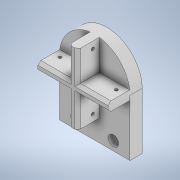
# Autodesk Inventor part: Test_Stand_Mounting_Plate
Saved by Autodesk Inventor 2022 (Build 260153000, 153)
## iProperties
Created: 2021-08-03
Part Number: Test_Stand_Mounting_Plate
Material: Generic
Document SubType Name: Modeling
Designer: exllu
Density: 1 g/cm^3
Appearance: Default
Author: exllu
Autodesk Inventor part; units mm, degrees
ref_plane "YZ Plane" through (0, 0, 0) normal (1, 0, 0) x (0, 1, 0)
ref_plane "XZ Plane" through (0, 0, 0) normal (0, 1, 0) x (-1, 0, 0)
ref_plane "XY Plane" through (0, 0, 0) normal (0, 0, 1) x (1, 0, 0)
sketch "Sketch1" plane through (0, 0, 0) normal (0, 0, 1) x (1, 0, 0)
  circle A0 centre (0, 0) radius 37.5
  line L0 (0, 0) -> (0, -25)
  circle A1 centre (0, -25) radius 3
  dimension "d0" = 75
  dimension "d1" = 25
  dimension "d2" = 6
  constraints: 2 centre point, 2 coincident, 2 end point, 1 vertical
  measures "d0" diameter of A0
  measures "d1" distance of L0.start L0.end
  measures "d2" diameter of A1
extrude "Extrusion1" add sketch "Sketch1" along normal blind 8 contours A0 | A1
sketch "Sketch2" plane through (0, 0, 8) normal (0, 0, 1) x (1, 0, 0)
  line L0 (0, 0) -> (17.6777, 17.6777)
  line L1 (0, 0) -> (25, 0) construction
  circle A0 centre (17.6777, 17.6777) radius 3.15
  circle A1 centre (-17.6777, 17.6777) radius 3.15
  circle A2 centre (-17.6777, -17.6777) radius 3.15
  circle A3 centre (17.6777, -17.6777) radius 3.15
  dimension "d5" = 25
  dimension "d6" = 45
  dimension "d7" = 6.3
  dimension "d10" = 360
  constraints: 4 centre point, 4 end point, 1 coincident, 1 equal length, 1 horizontal, 9 other
  measures "d5" distance of L0.start L0.end
  measures "d6" angle of L1 L0
  measures "d7" diameter of A0
extrude "Extrusion2" cut sketch "Sketch2" against normal blind 10
sketch "Sketch3" plane through (0, 0, 8) normal (0, 0, 1) x (1, 0, 0)
  arc A0 (-21.9203, 13.435) -> (-13.435, 21.9203) centre (-17.6777, 17.6777) ccw
  line L0 (-17.6777, 17.6777) -> (-11.6777, 17.6777) construction
  line L1 (-13.435, 21.9203) -> (-19.9189, 28.4042)
  line L2 (-21.9203, 13.435) -> (-28.4042, 19.9189)
  line L3 (-28.4042, 19.9189) -> (-19.9189, 28.4042)
  arc A1 (-13.435, -21.9203) -> (-21.9203, -13.435) centre (-17.6777, -17.6777) ccw
  line L4 (-17.6777, -17.6777) -> (-17.6777, -11.6777) construction
  line L5 (-21.9203, -13.435) -> (-28.4042, -19.9189)
  line L6 (-13.435, -21.9203) -> (-19.9189, -28.4042)
  line L7 (-19.9189, -28.4042) -> (-28.4042, -19.9189)
  arc A2 (21.9203, -13.435) -> (13.435, -21.9203) centre (17.6777, -17.6777) ccw
  line L8 (17.6777, -17.6777) -> (11.6777, -17.6777) construction
  line L9 (13.435, -21.9203) -> (19.9189, -28.4042)
  line L10 (21.9203, -13.435) -> (28.4042, -19.9189)
  line L11 (28.4042, -19.9189) -> (19.9189, -28.4042)
  arc A3 (13.435, 21.9203) -> (21.9203, 13.435) centre (17.6777, 17.6777) ccw
  line L12 (17.6777, 17.6777) -> (17.6777, 11.6777) construction
  line L13 (21.9203, 13.435) -> (28.4042, 19.9189)
  line L14 (13.435, 21.9203) -> (19.9189, 28.4042)
  line L15 (19.9189, 28.4042) -> (28.4042, 19.9189)
  circle A4 centre (0, 0) radius 31.5
  point P0 (-26.1087, 17.6234)
  point P1 (-26.1087, -17.6234)
  point P2 (-17.6234, -26.1087)
  point P3 (17.6234, -26.1087)
  point P4 (26.1087, -17.6234)
  point P5 (26.1087, 17.6234)
  point P6 (17.6234, 26.1087)
  point P7 (-17.6234, 26.1087)
  dimension "d14" = 12
  dimension "d18" = 360
  constraints: 32 end point, 8 point on circle, 5 centre point, 5 coincident, 2 tangent, 1 horizontal, 1 perpendicular, 49 other
  measures "d14" diameter of A0
sketch "Sketch4" plane through (0, 0, 0) normal (0, 0, -1) x (-1, 0, 0)
  circle A0 centre (0, 0) radius 42.8826
  constraints: 1 centre point, 1 coincident
extrude "Extrusion4" cut sketch "Sketch4" against normal blind 2
sketch "Sketch5" plane through (0, 0, 8) normal (0, 0, 1) x (1, 0, 0)
  line L0 (0, 0) -> (8, 0)
  line L1 (8, 0) -> (8, -40)
  line L2 (8, -40) -> (-8, -40)
  line L3 (-8, -40) -> (-8, 40)
  line L4 (-8, 40) -> (8, 40)
  line L5 (8, 40) -> (8, -40)
  line L6 (0, 0) -> (0, 8)
  line L7 (0, 8) -> (40, 8)
  line L8 (40, 8) -> (40, -8)
  line L9 (40, -8) -> (-40, -8)
  line L10 (-40, -8) -> (-40, 8)
  line L11 (-40, 8) -> (40, 8)
  line L12 (0, 0) -> (0, 40)
  line L13 (0, 40) -> (-5, 40)
  line L14 (-5, 40) -> (5, 40)
  line L15 (5, 40) -> (5, -40)
  line L16 (5, -40) -> (-5, -40)
  line L17 (-5, -40) -> (-5, 40)
  point P0 (8, -8)
  point P1 (8, 8)
  point P2 (-8, 8)
  point P3 (-8, -8)
  dimension "d24" = 8
  dimension "d25" = 40
  dimension "d26" = 16
  dimension "d27" = 80
  dimension "d30" = 90
  dimension "d34" = 5
  dimension "d35" = 10
  constraints: 36 end point, 4 parallel, 3 perpendicular, 2 coincident, 2 horizontal, 2 point on line, 1 midpoint, 12 other
  measures "d24" distance of L0.start L0.end
  measures "d25" distance of L0.end L1.end
  measures "d26" distance of L3.end L4.end
  measures "d27" distance of L2.end L3.end
  measures "d34" distance of L12.end L13.end
  measures "d35" distance of L15.end L16.end
sketch "Sketch6" plane through (0, 0, 8) normal (0, 0, 1) x (1, 0, 0)
  line L0 (0, 0) -> (0, 40)
  line L1 (0, 40) -> (-5, 40)
  line L2 (-5, 40) -> (5, 40)
  line L3 (5, 40) -> (5, -40)
  line L4 (5, -40) -> (-5, -40)
  line L5 (-5, -40) -> (-5, 40)
  line L6 (0, 0) -> (-40, 0)
  line L7 (-40, 0) -> (-40, -5)
  line L8 (-40, -5) -> (-40, 5)
  line L9 (-40, 5) -> (40, 5)
  line L10 (40, 5) -> (40, -5)
  line L11 (40, -5) -> (-40, -5)
  circle A0 centre (0, 0) radius 37.5
  point P0 (5, -5)
  point P1 (5, 5)
  point P2 (-5, 5)
  point P3 (-5, -5)
  point P4 (37.1652, 5)
  point P5 (5, 37.1652)
  point P6 (-5, 37.1652)
  point P7 (-37.1652, 5)
  point P8 (-37.1652, -5)
  point P9 (-5, -37.1652)
  point P10 (5, -37.1652)
  point P11 (37.1652, -5)
  dimension "d36" = 40
  dimension "d37" = 5
  dimension "d38" = 10
  dimension "d39" = 80
  dimension "d42" = 90
  dimension "d46" = 75
  constraints: 24 end point, 2 coincident, 2 parallel, 2 perpendicular, 1 centre point, 1 horizontal, 1 vertical, 12 other
  measures "d36" distance of L0.start L0.end
  measures "d37" distance of L0.end L1.end
  measures "d38" distance of L3.end L4.end
  measures "d39" distance of L2.end L3.end
  measures "d46" diameter of A0
extrude "Extrusion7" add sketch "Sketch6" along normal blind 30 contours L6 L5 L9 L0 | L0 L9 L3 L11 L5 L6 | L9 L5 A0 L0 | L0 A0 L3 L9 | L6 A0 L9 L5 | L5 L11 A0 L6 | L9 A0 L11 L3 | L11 L3 A0 L5
sketch "Sketch7" plane through (5, 5, 8) normal (0, 1, 0) x (1, 0, 0)
  line L0 (0, 0) -> (0, -30) projected
  line L1 (0, 0) -> (-5, 0)
  line L2 (-5, 0) -> (25, 0)
  line L3 (0, 0) -> (32.1652, 0) projected
  line L4 (25, 0) -> (25, -14)
  circle A0 centre (25, -14) radius 1.65
  point P0 (-5, 8)
  dimension "d49" = 5
  dimension "d50" = 30
  dimension "d51" = 14
  dimension "d52" = 3.3
  constraints: 6 end point, 1 centre point, 1 coincident, 1 horizontal, 1 point on line, 1 vertical
  measures "d49" distance of L0.start L1.end
  measures "d50" distance of L1.end L2.end
  measures "d51" distance of L2.end L4.end
  measures "d52" diameter of A0
extrude "Extrusion8" cut sketch "Sketch7" against normal blind 20
ref_plane "Work Plane1" through (5, 0, 8) normal (0, 1, 0) x (1, 0, 0)
ref_plane "Work Plane2" through (0, 5, 8) normal (1, 0, 0) x (0, 0, -1)
pattern_circular "Circular Pattern2" count 2 over 90 about axis through (0, 0, 8) along (0, 0, 1) of "Extrusion8"
sketch "Sketch8" plane through (-37.1652, 5, 8) normal (0, 1, 0) x (1, 0, 0)
  line L0 (32.1652, 0) -> (32.1652, -30) projected
  line L1 (32.1652, 0) -> (37.1652, 0)
  line L2 (37.1652, 0) -> (5.9902, 0)
  line L3 (22.6375, 0) -> (16.3375, 0) projected
  line L4 (5.9902, 0) -> (5.9902, -14)
  circle A0 centre (5.9902, -14) radius 2.15
  point P0 (37.1652, 8)
  dimension "d61" = 31.175
  dimension "d62" = 14
  dimension "d63" = 4.3
  constraints: 6 end point, 1 centre point, 1 coincident, 1 collinear, 1 horizontal, 1 perpendicular
  measures "d61" distance of L1.end L2.end
  measures "d62" distance of L2.end L4.end
  measures "d63" diameter of A0
extrude "Extrusion9" [suppressed]
pattern_circular "Circular Pattern3" count 2 over 360 about axis through (0, 0, 8) along (0, 0, -1) of "Extrusion8"
sketch "Sketch10" plane through (5, 5, 8) normal (1, 0, 0) x (0, 0, -1)
  line L0 (0, 0) -> (-30, 0) projected
  line L1 (0, 0) -> (-30, 0)
  line L2 (-30, 0) -> (-30, 35.3175)
  line L3 (-30, 35.3175) -> (0, 35.3175)
  line L4 (0, 35.3175) -> (0, 0)
  line L5 (0, -10) -> (-30, -10) projected
  line L6 (0, -10) -> (-32.3439, -10)
  line L7 (-32.3439, -10) -> (-32.3439, -45.8466)
  line L8 (-32.3439, -45.8466) -> (0, -45.8466)
  line L9 (0, -45.8466) -> (0, -10)
  point P0 (8, -5)
  constraints: 16 end point, 4 parallel, 2 horizontal, 2 perpendicular
extrude "Extrusion11" cut sketch "Sketch10" against normal blind 0.12
mirror "Mirror2" about plane through (0, 5, 8) normal (1, 0, 0) of "Extrusion11"
sketch "Sketch11" plane through (37.1652, 5, 38) normal (0, 1, 0) x (1, 0, 0)
  line L0 (-32.2852, 30) -> (-32.2852, 0) projected
  line L1 (-32.2852, 30) -> (5.1404, 30)
  line L2 (5.1404, 30) -> (5.1404, -1.2125)
  line L3 (5.1404, -1.2125) -> (-32.2852, -1.2125)
  line L4 (-32.2852, -1.2125) -> (-32.2852, 30)
  line L5 (-74.3303, 30) -> (-42.0452, 30) projected
  line L6 (-42.0452, 30) -> (-76.613, 30)
  line L7 (-76.613, 30) -> (-76.613, -1.2125)
  line L8 (-76.613, -1.2125) -> (-42.0452, -1.2125)
  line L9 (-42.0452, -1.2125) -> (-42.0452, 30)
  point P0 (-37.1652, 38)
  constraints: 16 end point, 4 parallel, 2 horizontal, 2 perpendicular, 1 point on line
extrude "Extrusion12" cut sketch "Sketch11" against normal blind 0.12
mirror "Mirror3" about plane through (5, 0, 8) normal (0, 1, 0) of "Extrusion12"
mirror "Mirror4" about plane through (5, 0, 8) normal (0, 1, 0) of "Extrusion8", "Circular Pattern2"
chamfer "Chamfer4" distance 3 angle 45 8 edges at (21.0306, 4.88, 38) (-21.0306, 4.88, 38) (4.88, -21.0306, 38) (4.88, 21.0306, 38) (-4.88, -21.0306, 38) (-4.88, 21.0306, 38) (21.0306, -4.88, 38) (-21.0306, -4.88, 38)
sketch "Sketch13" plane through (0, 0, 8) normal (0, 0, 1) x (1, 0, 0)
  arc A0 (37.1811, 4.88) -> (4.88, 37.1811) centre (0, 0) ccw projected
  circle A1 centre (0, 0) radius 37.5
  line L0 (37.1811, 4.88) -> (4.88, 4.88) projected
  line L1 (4.88, 4.88) -> (4.88, 37.1811) projected
  line L2 (37.1811, 4.88) -> (4.88, 4.88)
  line L3 (4.88, 4.88) -> (4.88, 37.1811)
  line L4 (4.88, 37.1811) -> (37.1811, 37.1811)
  line L5 (37.1811, 37.1811) -> (37.1811, 4.88)
  circle A2 centre (17.6777, 17.6777) radius 3.15 projected
  circle A3 centre (17.6777, 17.6777) radius 6
  line L6 (0, 0) -> (0, 7.2893)
  line L7 (0, 0) -> (7.7636, 0)
  arc A4 (-4.88, 37.1811) -> (-37.1811, 4.88) centre (0, 0) ccw
  circle A5 centre (0, 0) radius 37.5
  line L8 (-37.1811, 4.88) -> (-4.88, 4.88)
  line L9 (-4.88, 4.88) -> (-4.88, 37.1811)
  line L10 (-37.1811, 4.88) -> (-4.88, 4.88)
  line L11 (-4.88, 4.88) -> (-4.88, 37.1811)
  line L12 (-4.88, 37.1811) -> (-37.1811, 37.1811)
  line L13 (-37.1811, 37.1811) -> (-37.1811, 4.88)
  circle A6 centre (-17.6777, 17.6777) radius 3.15
  circle A7 centre (-17.6777, 17.6777) radius 6
  arc A8 (4.88, -37.1811) -> (37.1811, -4.88) centre (0, 0) ccw
  circle A9 centre (0, 0) radius 37.5
  line L14 (37.1811, -4.88) -> (4.88, -4.88)
  line L15 (4.88, -4.88) -> (4.88, -37.1811)
  line L16 (37.1811, -4.88) -> (4.88, -4.88)
  line L17 (4.88, -4.88) -> (4.88, -37.1811)
  line L18 (4.88, -37.1811) -> (37.1811, -37.1811)
  line L19 (37.1811, -37.1811) -> (37.1811, -4.88)
  circle A10 centre (17.6777, -17.6777) radius 3.15
  circle A11 centre (17.6777, -17.6777) radius 6
  line L20 (0, 0) -> (0, -7.2893)
  arc A12 (-37.1811, -4.88) -> (-4.88, -37.1811) centre (0, 0) ccw
  circle A13 centre (0, 0) radius 37.5
  line L21 (-37.1811, -4.88) -> (-4.88, -4.88)
  line L22 (-4.88, -4.88) -> (-4.88, -37.1811)
  line L23 (-37.1811, -4.88) -> (-4.88, -4.88)
  line L24 (-4.88, -4.88) -> (-4.88, -37.1811)
  line L25 (-4.88, -37.1811) -> (-37.1811, -37.1811)
  line L26 (-37.1811, -37.1811) -> (-37.1811, -4.88)
  circle A14 centre (-17.6777, -17.6777) radius 3.15
  circle A15 centre (-17.6777, -17.6777) radius 6
  arc A16 (1.88, 37.4528) -> (-1.88, 37.4528) centre (0, 0) ccw projected
  line L27 (1.88, 37.4528) -> (-1.88, 37.4528)
  line L28 (4.88, 37.1811) -> (17.88, 37.1811)
  line L29 (4.88, 37.1811) -> (4.88, 24.0161)
  point P0 (-37.1811, -4.88)
  dimension "d96" = 12
  dimension "d97" = 13
  dimension "d98" = 13.165
  constraints: 56 end point, 22 symmetric about line, 11 centre point, 7 point on circle, 5 coincident, 4 horizontal, 2 line through centre, 2 parallel, 2 point on line, 1 perpendicular, 1 vertical, 18 other
  measures "d96" diameter of A3
  measures "d97" distance of L1.end L28.end
  measures "d98" distance of L1.end L29.end
extrude "Extrusion14" add sketch "Sketch13" along normal blind 7 contours L0 L1 A0 | A1 L15 L14 | L9 L8 A1 | A1 L21 L22
sketch "Sketch19" plane through (0, 0, 2) normal (0, 0, -1) x (-1, 0, 0)
  circle A0 centre (-17.6777, 17.6777) radius 3.15 projected
  circle A1 centre (-17.6777, 17.6777) radius 9.67
  circle A2 centre (17.6777, 17.6777) radius 3.15 projected
  circle A3 centre (17.6777, 17.6777) radius 9.0628
  circle A4 centre (17.6777, -17.6777) radius 3.15 projected
  circle A5 centre (17.6777, -17.6777) radius 10.6824
  circle A6 centre (-17.6777, -17.6777) radius 3.15 projected
  circle A7 centre (-17.6777, -17.6777) radius 10.6824
  point P0 (0, 0)
  constraints: 4 centre point, 4 coincident
extrude "Extrusion19" add sketch "Sketch19" against normal blind 13 contours A0 | A1 | A2 | A3 | A4 | A5 | A6 | A7
sketch "Sketch21" plane through (0, 0, 2) normal (0, 0, -1) x (-1, 0, 0)
  circle A0 centre (0, 0) radius 37.5 projected
  line L0 (-37.5, 0) -> (37.5, 0)
  line L1 (37.5, 0) -> (37.5, -60)
  line L2 (37.5, -60) -> (-37.5, -60)
  line L3 (-37.5, -60) -> (-37.5, 0)
  dimension "d145" = 75
  dimension "d146" = 60
  constraints: 8 end point, 2 parallel, 1 horizontal, 1 perpendicular, 2 other
  measures "d145" distance of L1.end L2.end
  measures "d146" distance of L0.end L1.end
extrude "Extrusion22" add sketch "Sketch21" against normal blind 13 contours L1 L2 L3 A0
sketch "Sketch22" plane through (0, 0, 15) normal (0, 0, 1) x (1, 0, 0)
  line L0 (0, 0) -> (20, 0)
  line L1 (20, 0) -> (20, -4.88)
  line L2 (4.88, -4.88) -> (37.1811, -4.88) projected
  line L3 (20, -4.88) -> (20, -10.38)
  line L4 (0, 0) -> (-20, 0)
  line L5 (-20, 0) -> (-20, -4.88)
  line L6 (-37.1811, -4.88) -> (-4.88, -4.88) projected
  line L7 (-20, -4.88) -> (-20, -10.38)
  line L8 (-20, -10.38) -> (20, -10.38)
  line L9 (20, -10.38) -> (20, -50.38)
  line L10 (20, -50.38) -> (-20, -50.38)
  line L11 (-20, -50.38) -> (-20, -10.38)
  circle A0 centre (-20, -50.38) radius 2.65
  circle A1 centre (-20, -10.38) radius 2.65
  circle A2 centre (20, -10.38) radius 2.65
  circle A3 centre (20, -50.38) radius 2.65
  dimension "d149" = 20
  dimension "d150" = 5.5
  dimension "d151" = 20
  dimension "d152" = 5.5
  dimension "d153" = 40
  dimension "d154" = 40
  dimension "d155" = 5.3
  dimension "d156" = 5.3
  dimension "d157" = 5.3
  dimension "d158" = 5.3
  constraints: 20 end point, 5 coincident, 4 centre point, 4 point on line, 3 horizontal, 3 perpendicular, 2 parallel
  measures "d149" distance of L0.start L0.end
  measures "d150" distance of L1.end L3.end
  measures "d151" distance of L0.start L4.end
  measures "d152" distance of L5.end L7.end
  measures "d153" distance of L9.end L10.end
  measures "d154" distance of L8.end L9.end
  measures "d155" diameter of A0
  measures "d156" diameter of A1
  measures "d157" diameter of A2
  measures "d158" diameter of A3
extrude "Extrusion23" cut sketch "Sketch22" against normal blind 13 contours A2 L9 L3 | L3 L8 A2 | A1 L8 L7 | L7 L11 A1 | L9 A2 L8 | L8 A1 L11 | A0 L10 L11 | L11 L10 A0 | A3 L10 L9 | L9 L10 A3
sketch "Sketch23" plane through (0, 0, 15) normal (0, 0, 1) x (1, 0, 0)
  circle A0 centre (-20, -10.38) radius 2.65 projected
  circle A1 centre (-20, -10.38) radius 5.5
  line L0 (-37.1811, -4.88) -> (-4.88, -4.88) projected
  circle A2 centre (20, -10.38) radius 2.65 projected
  circle A3 centre (20, -10.38) radius 5.5
  circle A4 centre (20, -50.38) radius 2.65 projected
  circle A5 centre (20, -50.38) radius 5.5
  circle A6 centre (-20, -50.38) radius 2.65 projected
  circle A7 centre (-20, -50.38) radius 5.5
  point P0 (0, 0)
  dimension "d161" = 11
  dimension "d162" = 11
  constraints: 4 centre point, 4 coincident, 1 tangent
  measures "d161" diameter of A5
  measures "d162" diameter of A7
extrude "Extrusion24" cut sketch "Sketch23" against normal blind 9 contours A0 | A1 | A3 | A4 | A5 | A6 | A7
body "Solid1"
